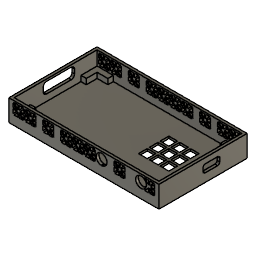
HomecurrentMoniter_BottomPlateHCM updated (Autodesk Fusion 360 design; units mm, degrees)
part number: 2026-06-16-14-03-26-042
Autodesk Fusion 360 part; units mm, degrees
note: some values were not read from the file. Set by a fixed rule: which sketch regions a step uses.
(part 1 of 2)
sketch "Sketch1" plane through (0, 0, 0) normal (0, 0, 1) x (1, 0, 0)
  line L0 (58.46, -118.98) -> (188.61, -118.98)
  line L1 (188.61, -118.98) -> (188.61, -46.12)
  line L2 (188.61, -46.12) -> (58.46, -46.12)
  line L3 (58.46, -46.12) -> (58.46, -118.98)
  line L4 (190.61, -121) -> (190.61, -44.12)
  line L5 (190.61, -44.12) -> (56.46, -44.12)
  line L6 (56.46, -44.12) -> (56.46, -120.98)
  line L7 (53.96, -123.48) -> (193.11, -123.48)
  line L8 (193.11, -123.48) -> (193.11, -41.62)
  line L9 (193.11, -41.62) -> (53.96, -41.62)
  line L10 (53.96, -41.62) -> (53.96, -123.48)
  line L11 (56.46, -44.12) -> (190.61, -44.12)
  line L12 (190.61, -44.12) -> (190.61, -121)
  line L13 (56.46, -120.98) -> (56.46, -44.12)
  line L14 (56.46, -44.12) -> (71.46, -44.12)
  line L15 (56.46, -59.12) -> (56.46, -44.12)
  line L16 (190.61, -44.12) -> (175.61, -44.12)
  line L17 (190.61, -59.12) -> (190.61, -44.12)
  line L18 (71.46, -120.98) -> (71.46, -115.98)
  line L19 (61.46, -105.98) -> (56.46, -105.98)
  line L20 (61.46, -115.98) -> (66.46, -115.98)
  line L21 (61.46, -110.98) -> (61.46, -115.98)
  line L22 (61.46, -110.98) -> (61.46, -105.98)
  line L23 (66.46, -115.98) -> (71.46, -115.98)
  line L24 (56.46, -120.98) -> (190.61, -120.98)
  line L25 (180.61, -115.98) -> (175.61, -115.98)
  line L26 (185.61, -115.98) -> (180.61, -115.98)
  line L27 (185.61, -105.98) -> (190.61, -105.98)
  line L28 (185.61, -110.98) -> (185.61, -115.98)
  line L29 (185.61, -110.98) -> (185.61, -105.98)
  line L30 (175.61, -120.98) -> (175.61, -115.98)
  line L31 (175.61, -44.12) -> (175.61, -49.12)
  line L32 (180.61, -49.12) -> (175.61, -49.12)
  line L33 (185.61, -49.12) -> (180.61, -49.12)
  line L34 (185.61, -54.12) -> (185.61, -49.12)
  line L35 (185.61, -54.12) -> (185.61, -59.12)
  line L36 (185.61, -59.12) -> (190.61, -59.12)
  line L37 (71.46, -44.12) -> (71.46, -49.12)
  line L38 (66.46, -49.12) -> (71.46, -49.12)
  line L39 (61.46, -49.12) -> (66.46, -49.12)
  line L40 (61.46, -54.12) -> (61.46, -49.12)
  line L41 (61.46, -54.12) -> (61.46, -59.12)
  line L42 (61.46, -59.12) -> (56.46, -59.12)
  point P0 (190.61, -120.98)
  point P1 (188.61, -118.98)
  point P2 (190.61, -120.98)
  dimension "d3" = 15
  dimension "d4" = 15
  dimension "d5" = 15
  dimension "d6" = 15
  dimension "d7" = 15
  dimension "d8" = 15
  constraint horizontal L11
  constraint vertical L12
  constraint vertical L13
  constraint horizontal L14
  constraint vertical L15
  constraint horizontal L16
  constraint vertical L17
  constraint vertical L18
  constraint horizontal L19
  constraint perpendicular L19 L22
  constraint perpendicular L18 L23
  constraint coincident L24 L30.start
  constraint perpendicular L24 L30
  constraint coincident L18.start L24
  constraint perpendicular L18 L24
  measures "d3" distance of L5.end L14.end
  measures "d4" distance of L5.end L15.start
  measures "d5" distance of L4.end L16.end
  measures "d6" distance of L4.end L17.start
  measures "d7" distance of L6.end L18.start
  measures "d8" distance of L6.end L19.end
extrude "Extrude1" add sketch "Sketch1" along normal blind 2 contours L0 L3 L18 L19 L20 L21 L22 L23 | L0 L3 L6 L13 L18 L19 L24 | L0 L1 L2 L3 L18 L19 L20 L21 L22 L23 L25 L26 L27 L28 L29 L30 L31 L32 L33 L34 L35 L36 L37 L38 L39 L40 L41 L42 | L0 L18 L24 L30 | L3 L6 L13 L19 L42 | L0 L1 L25 L26 L27 L28 L29 L30 | L0 L1 L4 L12 L24 L27 L30 | L2 L3 L5 L6 L11 L13 L14 L15 L37 L42 | L2 L3 L37 L38 L39 L40 L41 L42 | L1 L4 L12 L27 L36 | L2 L5 L11 L31 L37 | L1 L2 L31 L32 L33 L34 L35 L36 | L1 L2 L4 L5 L11 L12 L16 L17 L31 L36 | L7 L8 L9 L10
extrude "Extrude2" add sketch "Sketch1" along normal blind 30
extrude "Extrude3" add 1 faces at (145.8933, -42.4533, 30) along direction (0, 0, -1) blind 6
extrude "Extrude4" add sketch "Sketch1" along normal blind 7 contours L0 L3 L18 L19 L20 L21 L22 L23 | L0 L1 L25 L26 L27 L28 L29 L30 | L2 L3 L5 L6 L11 L13 L14 L15 L37 L42 | L2 L3 L37 L38 L39 L40 L41 L42 | L1 L2 L31 L32 L33 L34 L35 L36 | L1 L2 L4 L5 L11 L12 L16 L17 L31 L36
sketch "Sketch2" plane through (0, 0, 0) normal (0, 0, 1) x (1, 0, 0)
extrude "Extrude5" add sketch "Sketch1" along normal blind 7 contours L0 L3 L6 L13 L18 L19 L24
extrude "Extrude6" add sketch "Sketch1" along normal blind 7 contours L0 L1 L25 L26 L27 L28 L29 L30 | L0 L1 L4 L12 L24 L27 L30
sketch "Sketch3" plane through (193.11, 0, 0) normal (1, 0, 0) x (0, 1, 0)
  line L0 (-123.48, 0) -> (-41.62, 0)
  line L1 (-41.62, 0) -> (-41.62, 30)
  line L2 (-123.48, 30) -> (-123.48, 0)
  line L3 (-77.8135, 12.9716) -> (-71.4735, 12.9716)
  line L4 (-71.4735, 12.9716) -> (-77.8135, 12.9716)
  arc A0 (-77.8135, 12.9716) -> (-79.1135, 11.6716) centre (-77.8135, 11.6716) ccw
  arc A1 (-77.8135, 12.9716) -> (-79.1135, 11.6716) centre (-77.8135, 11.6716) ccw
  arc A2 (-70.1735, 11.6716) -> (-71.4735, 12.9716) centre (-71.4735, 11.6716) ccw
  arc A3 (-70.1735, 11.6716) -> (-71.4735, 12.9716) centre (-71.4735, 11.6716) ccw
  line L5 (-70.1735, 11.6716) -> (-70.1735, 11.1116)
  line L6 (-70.1735, 11.1116) -> (-70.1735, 11.1366)
  line L7 (-70.1735, 11.1366) -> (-70.1735, 11.1116)
  line L8 (-70.1735, 11.1116) -> (-70.1735, 11.1366)
  line L9 (-70.1735, 11.1366) -> (-70.1735, 11.3916)
  line L10 (-70.1735, 11.3916) -> (-70.1735, 11.6716)
  line L11 (-79.1135, 11.1116) -> (-79.1135, 11.6716)
  line L12 (-79.1135, 11.6716) -> (-79.1135, 11.3916)
  line L13 (-79.1135, 11.3916) -> (-79.1135, 11.1366)
  line L14 (-79.1135, 11.1366) -> (-79.1135, 11.1116)
  line L15 (-79.1135, 11.1116) -> (-79.1135, 11.1366)
  line L16 (-79.1135, 11.1366) -> (-79.1135, 11.1116)
  arc A4 (-79.1135, 11.1116) -> (-77.8135, 9.8116) centre (-77.8135, 11.1116) ccw
  arc A5 (-79.1135, 11.1116) -> (-77.8135, 9.8116) centre (-77.8135, 11.1116) ccw
  arc A6 (-71.4735, 9.8116) -> (-70.1735, 11.1116) centre (-71.4735, 11.1116) ccw
  arc A7 (-71.4735, 9.8116) -> (-70.1735, 11.1116) centre (-71.4735, 11.1116) ccw
  line L17 (-80.5, 15) -> (-68.9871, 15)
  line L18 (-66.9871, 13) -> (-66.9871, 9.8116)
  line L19 (-68.9871, 7.8116) -> (-80.5, 7.8116)
  line L20 (-82.5, 9.8116) -> (-82.5, 13)
  arc A8 (-66.9871, 13) -> (-68.9871, 15) centre (-68.9871, 13) ccw
  arc A9 (-68.9871, 7.8116) -> (-66.9871, 9.8116) centre (-68.9871, 9.8116) ccw
  arc A10 (-82.5, 9.8116) -> (-80.5, 7.8116) centre (-80.5, 9.8116) ccw
  arc A11 (-80.5, 15) -> (-82.5, 13) centre (-80.5, 13) ccw
  line L21 (-41.62, 30) -> (-123.48, 30)
  dimension "d24" = 2
  constraint horizontal L17
  constraint vertical L18
  constraint horizontal L19
  constraint vertical L20
  constraint tangent L17 A8
  constraint tangent L18 A8
  constraint tangent L18 A9
  constraint tangent L19 A9
  constraint equal A8 A9
  constraint tangent L19 A10
  constraint tangent L20 A10
  constraint equal A8 A10
  constraint tangent L17 A11
  constraint tangent L20 A11
  constraint equal A8 A11
  measures "d24" radius of A8
extrude "Extrude7" cut sketch "Sketch3" against normal up to surface (2.5 mm away) contours L17 L18 L19 L20 A8 A9 A10 A11
sketch "Sketch4" plane through (53.96, 0, 0) normal (-1, 0, 0) x (0, -1, 0)
  line L0 (41.62, 0) -> (123.48, 0)
  line L1 (123.48, 0) -> (123.48, 30)
  line L2 (41.62, 30) -> (41.62, 0)
  arc A0 (87.1797, 12.5216) -> (87.0797, 12.6216) centre (87.0797, 12.5216) ccw
  line L3 (87.1797, 10.4716) -> (87.1797, 12.5216)
  line L4 (87.3797, 10.4716) -> (87.1797, 10.4716)
  line L5 (87.3797, 10.4216) -> (87.3797, 10.4716)
  line L6 (88.3797, 10.4216) -> (87.3797, 10.4216)
  line L7 (88.3797, 10.3216) -> (88.3797, 10.4216)
  line L8 (88.3797, 9.5216) -> (88.3797, 10.3216)
  line L9 (85.3997, 9.5216) -> (88.3797, 9.5216)
  line L10 (85.3997, 9.5216) -> (85.3947, 9.5216)
  line L11 (85.3947, 9.5216) -> (85.2997, 9.5216)
  line L12 (84.7997, 9.5216) -> (85.2997, 9.5216)
  line L13 (84.7997, 9.5216) -> (84.7948, 9.5216)
  line L14 (84.7948, 9.5216) -> (84.6997, 9.5216)
  line L15 (84.1297, 9.5216) -> (84.6997, 9.5216)
  line L16 (84.1297, 9.5216) -> (84.1247, 9.5216)
  line L17 (84.1247, 9.5216) -> (84.0297, 9.5216)
  line L18 (83.5297, 9.5216) -> (84.0297, 9.5216)
  line L19 (83.5297, 9.5216) -> (83.5248, 9.5216)
  line L20 (83.5248, 9.5216) -> (83.4297, 9.5216)
  line L21 (82.8597, 9.5216) -> (83.4297, 9.5216)
  line L22 (82.8597, 9.5216) -> (82.8547, 9.5216)
  line L23 (82.8547, 9.5216) -> (82.7597, 9.5216)
  line L24 (82.2597, 9.5216) -> (82.7597, 9.5216)
  line L25 (82.2597, 9.5216) -> (82.2548, 9.5216)
  line L26 (82.2548, 9.5216) -> (82.1597, 9.5216)
  line L27 (81.5897, 9.5216) -> (82.1597, 9.5216)
  line L28 (81.5897, 9.5216) -> (81.5847, 9.5216)
  line L29 (81.5847, 9.5216) -> (81.4897, 9.5216)
  line L30 (80.9897, 9.5216) -> (81.4897, 9.5216)
  line L31 (80.9897, 9.5216) -> (80.9848, 9.5216)
  line L32 (80.9848, 9.5216) -> (80.8897, 9.5216)
  line L33 (80.3197, 9.5216) -> (80.8897, 9.5216)
  line L34 (80.3197, 9.5216) -> (80.3147, 9.5216)
  line L35 (80.3147, 9.5216) -> (80.2197, 9.5216)
  line L36 (79.7197, 9.5216) -> (80.2197, 9.5216)
  line L37 (79.7197, 9.5216) -> (79.7148, 9.5216)
  line L38 (79.7148, 9.5216) -> (79.6197, 9.5216)
  line L39 (79.0497, 9.5216) -> (79.6197, 9.5216)
  line L40 (79.0497, 9.5216) -> (79.0447, 9.5216)
  line L41 (79.0447, 9.5216) -> (78.9497, 9.5216)
  line L42 (78.4497, 9.5216) -> (78.9497, 9.5216)
  line L43 (78.4497, 9.5216) -> (78.4448, 9.5216)
  line L44 (78.4448, 9.5216) -> (78.3497, 9.5216)
  line L45 (77.7797, 9.5216) -> (78.3497, 9.5216)
  line L46 (77.7797, 9.5216) -> (77.7747, 9.5216)
  line L47 (77.7747, 9.5216) -> (77.6797, 9.5216)
  line L48 (77.1797, 9.5216) -> (77.6797, 9.5216)
  line L49 (77.1797, 9.5216) -> (77.1748, 9.5216)
  line L50 (77.1748, 9.5216) -> (77.0797, 9.5216)
  line L51 (76.5097, 9.5216) -> (77.0797, 9.5216)
  line L52 (76.5097, 9.5216) -> (76.5047, 9.5216)
  line L53 (76.5047, 9.5216) -> (76.4097, 9.5216)
  line L54 (75.9097, 9.5216) -> (76.4097, 9.5216)
  line L55 (75.9097, 9.5216) -> (75.9048, 9.5216)
  line L56 (75.9048, 9.5216) -> (75.8097, 9.5216)
  line L57 (75.2397, 9.5216) -> (75.8097, 9.5216)
  line L58 (75.2397, 9.5216) -> (75.2347, 9.5216)
  line L59 (75.2347, 9.5216) -> (75.1397, 9.5216)
  line L60 (74.6397, 9.5216) -> (75.1397, 9.5216)
  line L61 (74.6397, 9.5216) -> (74.6348, 9.5216)
  line L62 (74.6348, 9.5216) -> (74.5397, 9.5216)
  line L63 (73.9697, 9.5216) -> (74.5397, 9.5216)
  line L64 (73.9697, 9.5216) -> (73.9647, 9.5216)
  line L65 (73.9647, 9.5216) -> (73.8697, 9.5216)
  line L66 (73.3697, 9.5216) -> (73.8697, 9.5216)
  line L67 (73.3697, 9.5216) -> (73.3648, 9.5216)
  line L68 (73.3648, 9.5216) -> (73.2697, 9.5216)
  line L69 (70.3797, 9.5216) -> (73.2697, 9.5216)
  line L70 (70.3797, 9.5216) -> (70.3797, 10.3216)
  line L71 (70.3797, 10.3216) -> (70.3797, 10.4216)
  line L72 (70.3797, 10.4216) -> (71.3797, 10.4216)
  line L73 (71.3797, 10.3216) -> (71.3797, 10.4216)
  line L74 (71.3797, 10.3216) -> (71.4797, 10.3216)
  line L75 (71.4797, 10.3216) -> (71.4797, 10.4216)
  line L76 (71.5797, 10.4216) -> (71.4797, 10.4216)
  line L77 (71.5797, 10.4216) -> (71.5797, 12.5216)
  arc A1 (71.6797, 12.6216) -> (71.5797, 12.5216) centre (71.6797, 12.5216) ccw
  line L78 (87.0797, 12.6216) -> (71.6797, 12.6216)
  line L79 (68, 18.0438) -> (91, 18.0438)
  line L80 (94, 15.0438) -> (94, 11)
  line L81 (91, 8) -> (68, 8)
  line L82 (65, 11) -> (65, 15.0438)
  arc A2 (68, 18.0438) -> (65, 15.0438) centre (68, 15.0438) ccw
  arc A3 (94, 15.0438) -> (91, 18.0438) centre (91, 15.0438) ccw
  arc A4 (91, 8) -> (94, 11) centre (91, 11) ccw
  arc A5 (65, 11) -> (68, 8) centre (68, 11) ccw
  line L83 (123.48, 30) -> (41.62, 30)
  dimension "d31" = 3
  constraint horizontal L79
  constraint vertical L80
  constraint horizontal L81
  constraint vertical L82
  constraint tangent L79 A2
  constraint tangent L82 A2
  constraint tangent L79 A3
  constraint tangent L80 A3
  constraint equal A2 A3
  constraint tangent L81 A4
  constraint tangent L80 A4
  constraint equal A2 A4
  constraint tangent L81 A5
  constraint tangent L82 A5
  constraint equal A2 A5
  measures "d31" radius of A2
extrude "Extrude8" cut sketch "Sketch4" against normal up to surface (2.5 mm away) contours A0 L3 L4 L5 L6 L7 L8 L9 L10 L11 L12 L13 L14 L15 L16 L17 L18 L19 L20 L21 L22 L23 L24 L25 L26 L27 L28 L29 L30 L31 L32 L33 L34 L35 L36 L37 L38 L39 L40 L41 L42 L43 L44 L45 L46 L47 L48 L49 L50 L51 L52 L53 L54 L55 L56 L57 L58 L59 L60 L61 L62 L63 L64 L65 L66 L67 L68 L69 L70 L71 L72 L73 L74 L75 L76 L77 A1 L78 | L79 L80 L81 L82 A2 A3 A4 A5
extrude "Extrude9" cut 1 faces at (145.8933, -42.4533, 30) along direction (0, 0, -1) blind 8
extrude "Extrude10" cut 1 faces at (145.8933, -42.4533, 22) along direction (0, 0, -1) blind 2
sketch "Sketch6" plane through (0, -123.48, 0) normal (0, -1, 0) x (1, 0, 0)
  line L0 (193.11, 20) -> (53.96, 20)
  line L1 (53.96, 20) -> (53.96, 0)
  line L2 (53.96, 0) -> (193.11, 0)
  line L3 (193.11, 0) -> (193.11, 20)
  line L4 (56.46, 20) -> (190.61, 20)
  line L5 (190.61, 20) -> (190.61, 7)
  line L6 (190.61, 7) -> (175.61, 7)
  line L7 (175.61, 7) -> (175.61, 2)
  line L8 (175.61, 2) -> (71.46, 2)
  line L9 (71.46, 2) -> (71.46, 7)
  line L10 (71.46, 7) -> (56.46, 7)
  line L11 (56.46, 7) -> (56.46, 20)
  line L12 (174.61, 3) -> (72.46, 3)
  line L13 (72.46, 3) -> (72.46, 8)
  line L14 (72.46, 8) -> (57.46, 8)
  line L15 (57.46, 8) -> (57.46, 19)
  line L16 (57.46, 19) -> (189.61, 19)
  line L17 (189.61, 19) -> (189.61, 8)
  line L18 (189.61, 8) -> (174.61, 8)
  line L19 (174.61, 8) -> (174.61, 3)
  line L20 (57.46, 19) -> (62.96, 19)
  line L21 (62.96, 19) -> (62.96, 13.5)
  line L22 (62.96, 13.5) -> (57.46, 13.5)
  line L23 (57.46, 13.5) -> (57.46, 19)
  line L24 (57.46, 19) -> (62.96, 13.5)
  line L25 (62.46, 18.5) -> (62.46, 14.7071)
  line L26 (58.6671, 18.5) -> (62.46, 14.7071)
  line L27 (58.6671, 18.5) -> (62.46, 18.5)
  line L28 (61.7529, 14) -> (57.96, 14)
  line L29 (57.96, 14) -> (57.96, 17.7929)
  line L30 (57.96, 17.7929) -> (61.7529, 14)
  line L31 (57.96, 13) -> (57.96, 9.2071)
  line L32 (57.96, 9.2071) -> (61.7529, 13)
  line L33 (61.7529, 13) -> (57.96, 13)
  line L34 (58.6671, 8.5) -> (62.46, 12.2929)
  line L35 (62.46, 8.5) -> (62.46, 12.2929)
  line L36 (58.6671, 8.5) -> (62.46, 8.5)
  line L37 (62.96, 13.5) -> (57.46, 13.5)
  line L38 (62.96, 8) -> (62.96, 13.5)
  line L39 (67.2529, 18.5) -> (63.46, 14.7071)
  line L40 (63.46, 18.5) -> (63.46, 14.7071)
  line L41 (67.2529, 18.5) -> (63.46, 18.5)
  line L42 (67.96, 17.7929) -> (64.1671, 14)
  line L43 (67.96, 14) -> (67.96, 17.7929)
  line L44 (64.1671, 14) -> (67.96, 14)
  line L45 (64.1671, 13) -> (67.96, 13)
  line L46 (67.96, 13) -> (67.96, 9.2071)
  line L47 (67.96, 9.2071) -> (64.1671, 13)
  line L48 (67.2529, 8.5) -> (63.46, 12.2929)
  line L49 (63.46, 8.5) -> (63.46, 12.2929)
  line L50 (67.2529, 8.5) -> (63.46, 8.5)
  line L51 (68.46, 8) -> (68.46, 19)
  line L52 (78.2529, 18.5) -> (74.46, 18.5)
  line L53 (78.2529, 18.5) -> (74.46, 14.7071)
  line L54 (74.46, 18.5) -> (74.46, 14.7071)
  line L55 (78.96, 17.7929) -> (75.1671, 14)
  line L56 (78.96, 14) -> (78.96, 17.7929)
  line L57 (75.1671, 14) -> (78.96, 14)
  line L58 (75.1671, 13) -> (78.96, 13)
  line L59 (78.96, 13) -> (78.96, 9.2071)
  line L60 (78.96, 9.2071) -> (75.1671, 13)
  line L61 (74.46, 8.5) -> (74.46, 12.2929)
  line L62 (78.2529, 8.5) -> (74.46, 12.2929)
  line L63 (78.2529, 8.5) -> (74.46, 8.5)
  line L64 (68.96, 17.7929) -> (72.7529, 14)
  line L65 (69.6671, 18.5) -> (73.46, 18.5)
  line L66 (68.96, 9.2071) -> (72.7529, 13)
  line L67 (73.46, 18.5) -> (73.46, 14.7071)
  line L68 (68.96, 13) -> (68.96, 9.2071)
  line L69 (69.6671, 18.5) -> (73.46, 14.7071)
  line L70 (72.7529, 14) -> (68.96, 14)
  line L71 (68.96, 14) -> (68.96, 17.7929)
  line L72 (72.7529, 13) -> (68.96, 13)
  line L73 (73.46, 8.5) -> (73.46, 12.2929)
  line L74 (69.6671, 8.5) -> (73.46, 12.2929)
  line L75 (69.6671, 8.5) -> (73.46, 8.5)
  line L76 (123.535, 19) -> (123.535, 3)
  line L77 (123.535, 19) -> (57.46, 19)
  line L78 (119.2421, 13) -> (123.035, 13)
  line L79 (107.535, 18.5) -> (107.535, 14.7071)
  line L80 (111.3279, 8.5) -> (107.535, 12.2929)
  line L81 (117.535, 18.5) -> (117.535, 14.7071)
  line L82 (123.535, 19) -> (118.035, 13.5)
  line L83 (117.535, 8.5) -> (117.535, 12.2929)
  line L84 (123.035, 9.2071) -> (119.2421, 13)
  line L85 (118.035, 13.5) -> (123.535, 13.5)
  line L86 (123.535, 19) -> (118.035, 19)
  line L87 (122.3279, 8.5) -> (118.535, 8.5)
  line L88 (122.3279, 18.5) -> (118.535, 14.7071)
  line L89 (123.035, 17.7929) -> (119.2421, 14)
  line L90 (106.535, 8.5) -> (106.535, 12.2929)
  line L91 (111.3279, 18.5) -> (107.535, 14.7071)
  line L92 (118.035, 19) -> (118.035, 13.5)
  line L93 (118.535, 18.5) -> (118.535, 14.7071)
  line L94 (112.035, 14) -> (112.035, 17.7929)
  line L95 (123.535, 13.5) -> (123.535, 19)
  line L96 (112.035, 17.7929) -> (108.2421, 14)
  line L97 (112.035, 9.2071) -> (108.2421, 13)
  line L98 (108.2421, 13) -> (112.035, 13)
  line L99 (123.035, 13) -> (123.035, 9.2071)
  line L100 (111.3279, 8.5) -> (107.535, 8.5)
  line L101 (105.8279, 13) -> (102.035, 13)
  line L102 (102.7421, 8.5) -> (106.535, 8.5)
  line L103 (105.8279, 14) -> (102.035, 14)
  line L104 (102.7421, 8.5) -> (106.535, 12.2929)
  line L105 (102.7421, 18.5) -> (106.535, 18.5)
  line L106 (102.035, 9.2071) -> (105.8279, 13)
  line L107 (102.035, 13) -> (102.035, 9.2071)
  line L108 (102.035, 17.7929) -> (105.8279, 14)
  line L109 (102.7421, 18.5) -> (106.535, 14.7071)
  line L110 (118.535, 8.5) -> (118.535, 12.2929)
  line L111 (113.035, 14) -> (113.035, 17.7929)
  line L112 (122.3279, 8.5) -> (118.535, 12.2929)
  line L113 (111.3279, 18.5) -> (107.535, 18.5)
  line L114 (113.035, 17.7929) -> (116.8279, 14)
  line L115 (122.3279, 18.5) -> (118.535, 18.5)
  line L116 (119.2421, 14) -> (123.035, 14)
  line L117 (107.535, 8.5) -> (107.535, 12.2929)
  line L118 (113.035, 13) -> (113.035, 9.2071)
  line L119 (106.535, 18.5) -> (106.535, 14.7071)
  line L120 (123.035, 14) -> (123.035, 17.7929)
  line L121 (113.7421, 18.5) -> (117.535, 18.5)
  line L122 (118.035, 13.5) -> (123.535, 13.5)
  line L123 (108.2421, 14) -> (112.035, 14)
  line L124 (112.035, 13) -> (112.035, 9.2071)
  line L125 (113.7421, 18.5) -> (117.535, 14.7071)
  line L126 (116.8279, 13) -> (113.035, 13)
  line L127 (113.7421, 8.5) -> (117.535, 8.5)
  line L128 (116.8279, 14) -> (113.035, 14)
  line L129 (102.035, 14) -> (102.035, 17.7929)
  line L130 (113.035, 9.2071) -> (116.8279, 13)
  line L131 (113.7421, 8.5) -> (117.535, 12.2929)
  line L132 (90.4975, 19) -> (84.9975, 19)
  line L133 (84.9975, 19) -> (84.9975, 13.5)
  line L134 (84.9975, 13.5) -> (90.4975, 13.5)
  line L135 (90.4975, 13.5) -> (90.4975, 19)
  line L136 (84.9975, 19) -> (90.4975, 13.5)
  line L137 (84.9975, 19) -> (90.4975, 19)
  line L138 (89.9975, 14.7071) -> (89.9975, 18.5)
  line L139 (89.9975, 18.5) -> (86.2046, 18.5)
  line L140 (86.2046, 18.5) -> (89.9975, 14.7071)
  line L141 (85.4975, 14) -> (85.4975, 17.7929)
  line L142 (85.4975, 17.7929) -> (89.2904, 14)
  line L143 (89.2904, 14) -> (85.4975, 14)
  line L144 (86.2046, 8.5) -> (89.9975, 12.2929)
  line L145 (89.9975, 8.5) -> (86.2046, 8.5)
  line L146 (89.9975, 12.2929) -> (89.9975, 8.5)
  line L147 (85.4975, 9.2071) -> (89.2904, 13)
  line L148 (85.4975, 13) -> (85.4975, 9.2071)
  line L149 (89.2904, 13) -> (85.4975, 13)
  line L150 (95.4975, 17.7929) -> (91.7046, 14)
  line L151 (95.4975, 14) -> (95.4975, 17.7929)
  line L152 (94.7904, 18.5) -> (90.9975, 14.7071)
  line L153 (90.9975, 18.5) -> (94.7904, 18.5)
  line L154 (90.9975, 14.7071) -> (90.9975, 18.5)
  line L155 (95.4975, 9.2071) -> (91.7046, 13)
  line L156 (90.9975, 12.2929) -> (90.9975, 8.5)
  line L157 (94.7904, 8.5) -> (90.9975, 12.2929)
  line L158 (95.4975, 13) -> (95.4975, 9.2071)
  line L159 (90.9975, 8.5) -> (94.7904, 8.5)
  line L160 (91.7046, 13) -> (95.4975, 13)
  line L161 (91.7046, 14) -> (95.4975, 14)
  line L162 (79, 19) -> (84.9975, 19)
  line L163 (168.11, 17.7929) -> (171.9029, 14)
  line L164 (168.8171, 18.5) -> (172.61, 14.7071)
  line L165 (168.8171, 8.5) -> (172.61, 12.2929)
  line L166 (123.535, 19) -> (189.61, 19)
  line L167 (171.9029, 14) -> (168.11, 14)
  line L168 (168.8171, 8.5) -> (172.61, 8.5)
  line L169 (171.9029, 13) -> (168.11, 13)
  line L170 (168.8171, 18.5) -> (172.61, 18.5)
  line L171 (168.11, 9.2071) -> (171.9029, 13)
  line L172 (144.3279, 18.5) -> (140.535, 18.5)
  line L173 (178.11, 14) -> (178.11, 17.7929)
  line L174 (157.0725, 8.5) -> (160.8654, 8.5)
  line L175 (173.61, 8.5) -> (173.61, 12.2929)
  line L176 (184.61, 18.5) -> (184.61, 14.7071)
  line L177 (151.5725, 13) -> (151.5725, 9.2071)
  line L178 (145.035, 9.2071) -> (141.2421, 13)
  line L179 (189.61, 19) -> (184.11, 19)
  line L180 (145.035, 17.7929) -> (141.2421, 14)
  line L181 (189.61, 13.5) -> (189.61, 19)
  line L182 (151.5725, 17.7929) -> (155.3654, 14)
  line L183 (156.0725, 14.7071) -> (156.0725, 18.5)
  line L184 (145.035, 13) -> (145.035, 9.2071)
  line L185 (188.4029, 8.5) -> (184.61, 8.5)
  line L186 (189.11, 9.2071) -> (185.3171, 13)
  line L187 (188.4029, 8.5) -> (184.61, 12.2929)
  line L188 (124.7421, 8.5) -> (128.535, 12.2929)
  line L189 (124.035, 9.2071) -> (127.8279, 13)
  line L190 (129.035, 19) -> (129.035, 13.5)
  line L191 (135.7421, 18.5) -> (139.535, 14.7071)
  line L192 (156.5725, 19) -> (162.0725, 19)
  line L193 (135.035, 13) -> (135.035, 9.2071)
  line L194 (139.535, 18.5) -> (139.535, 14.7071)
  line L195 (130.2421, 13) -> (134.035, 13)
  line L196 (157.0725, 12.2929) -> (157.0725, 8.5)
  line L197 (140.535, 18.5) -> (140.535, 14.7071)
  line L198 (183.61, 18.5) -> (183.61, 14.7071)
  line L199 (134.035, 9.2071) -> (130.2421, 13)
  line L200 (134.035, 13) -> (134.035, 9.2071)
  line L201 (185.3171, 14) -> (189.11, 14)
  line L202 (129.535, 8.5) -> (129.535, 12.2929)
  line L203 (184.11, 8) -> (184.11, 13.5)
  line L204 (157.0725, 14.7071) -> (157.0725, 18.5)
  line L205 (184.61, 8.5) -> (184.61, 12.2929)
  line L206 (185.3171, 13) -> (189.11, 13)
  line L207 (135.035, 17.7929) -> (138.8279, 14)
  line L208 (188.4029, 18.5) -> (184.61, 14.7071)
  line L209 (183.61, 8.5) -> (183.61, 12.2929)
  line L210 (128.535, 8.5) -> (128.535, 12.2929)
  line L211 (189.11, 17.7929) -> (185.3171, 14)
  line L212 (179.8171, 8.5) -> (183.61, 12.2929)
  line L213 (144.3279, 8.5) -> (140.535, 8.5)
  line L214 (179.8171, 8.5) -> (183.61, 8.5)
  line L215 (182.9029, 14) -> (179.11, 14)
  line L216 (179.11, 9.2071) -> (182.9029, 13)
  line L217 (179.11, 17.7929) -> (182.9029, 14)
  line L218 (123.535, 19) -> (129.035, 19)
  line L219 (144.3279, 18.5) -> (140.535, 14.7071)
  line L220 (144.3279, 8.5) -> (140.535, 12.2929)
  line L221 (156.0725, 18.5) -> (152.2796, 18.5)
  line L222 (156.0725, 8.5) -> (152.2796, 8.5)
  line L223 (179.8171, 18.5) -> (183.61, 14.7071)
  line L224 (155.3654, 14) -> (151.5725, 14)
  line L225 (177.4029, 8.5) -> (173.61, 12.2929)
  line L226 (141.2421, 13) -> (145.035, 13)
  line L227 (156.0725, 12.2929) -> (156.0725, 8.5)
  line L228 (160.8654, 18.5) -> (157.0725, 14.7071)
  line L229 (123.535, 13.5) -> (123.535, 19)
  line L230 (129.035, 13.5) -> (123.535, 13.5)
  line L231 (162.0725, 19) -> (162.0725, 13.5)
  line L232 (172.61, 18.5) -> (172.61, 14.7071)
  line L233 (178.11, 9.2071) -> (174.3171, 13)
  line L234 (151.5725, 9.2071) -> (155.3654, 13)
  line L235 (129.035, 13.5) -> (123.535, 13.5)
  line L236 (177.4029, 18.5) -> (173.61, 18.5)
  line L237 (157.0725, 18.5) -> (160.8654, 18.5)
  line L238 (124.7421, 18.5) -> (128.535, 14.7071)
  line L239 (124.035, 14) -> (124.035, 17.7929)
  line L240 (130.2421, 14) -> (134.035, 14)
  line L241 (135.7421, 8.5) -> (139.535, 8.5)
  line L242 (129.535, 18.5) -> (129.535, 14.7071)
  line L243 (124.035, 17.7929) -> (127.8279, 14)
  line L244 (128.535, 18.5) -> (128.535, 14.7071)
  line L245 (135.035, 9.2071) -> (138.8279, 13)
  line L246 (135.7421, 8.5) -> (139.535, 12.2929)
  line L247 (127.8279, 14) -> (124.035, 14)
  line L248 (134.035, 14) -> (134.035, 17.7929)
  line L249 (135.035, 14) -> (135.035, 17.7929)
  line L250 (139.535, 8.5) -> (139.535, 12.2929)
  line L251 (138.8279, 14) -> (135.035, 14)
  line L252 (140.535, 8.5) -> (140.535, 12.2929)
  line L253 (133.3279, 18.5) -> (129.535, 18.5)
  line L254 (124.035, 13) -> (124.035, 9.2071)
  line L255 (152.2796, 8.5) -> (156.0725, 12.2929)
  line L256 (182.9029, 13) -> (179.11, 13)
  line L257 (155.3654, 13) -> (151.5725, 13)
  line L258 (123.535, 19) -> (129.035, 13.5)
  line L259 (157.7796, 14) -> (161.5725, 14)
  line L260 (145.035, 14) -> (145.035, 17.7929)
  line L261 (161.5725, 9.2071) -> (157.7796, 13)
  line L262 (179.8171, 18.5) -> (183.61, 18.5)
  line L263 (151.5725, 14) -> (151.5725, 17.7929)
  line L264 (141.2421, 14) -> (145.035, 14)
  line L265 (156.5725, 13.5) -> (156.5725, 19)
  line L266 (152.2796, 18.5) -> (156.0725, 14.7071)
  line L267 (157.7796, 13) -> (161.5725, 13)
  line L268 (133.3279, 8.5) -> (129.535, 12.2929)
  line L269 (173.61, 18.5) -> (173.61, 14.7071)
  line L270 (179.11, 13) -> (179.11, 9.2071)
  line L271 (161.5725, 14) -> (161.5725, 17.7929)
  line L272 (178.61, 8) -> (178.61, 19)
  line L273 (160.8654, 8.5) -> (157.0725, 12.2929)
  line L274 (161.5725, 17.7929) -> (157.7796, 14)
  line L275 (179.11, 14) -> (179.11, 17.7929)
  line L276 (177.4029, 8.5) -> (173.61, 8.5)
  line L277 (184.11, 13.5) -> (189.61, 13.5)
  line L278 (188.4029, 18.5) -> (184.61, 18.5)
  line L279 (133.3279, 8.5) -> (129.535, 8.5)
  line L280 (124.7421, 18.5) -> (128.535, 18.5)
  line L281 (127.8279, 13) -> (124.035, 13)
  line L282 (162.0725, 19) -> (156.5725, 13.5)
  line L283 (178.11, 13) -> (178.11, 9.2071)
  line L284 (189.61, 19) -> (184.11, 13.5)
  line L285 (138.8279, 13) -> (135.035, 13)
  line L286 (172.61, 8.5) -> (172.61, 12.2929)
  line L287 (162.0725, 13.5) -> (156.5725, 13.5)
  line L288 (174.3171, 14) -> (178.11, 14)
  line L289 (184.11, 13.5) -> (189.61, 13.5)
  line L290 (162.0725, 19) -> (156.5725, 19)
  line L291 (177.4029, 18.5) -> (173.61, 14.7071)
  line L292 (168.07, 19) -> (162.0725, 19)
  line L293 (168.11, 14) -> (168.11, 17.7929)
  line L294 (174.3171, 13) -> (178.11, 13)
  line L295 (189.11, 14) -> (189.11, 17.7929)
  line L296 (161.5725, 13) -> (161.5725, 9.2071)
  line L297 (133.3279, 18.5) -> (129.535, 14.7071)
  line L298 (134.035, 17.7929) -> (130.2421, 14)
  line L299 (178.11, 17.7929) -> (174.3171, 14)
  line L300 (189.11, 13) -> (189.11, 9.2071)
  line L301 (135.7421, 18.5) -> (139.535, 18.5)
  line L302 (184.11, 19) -> (184.11, 13.5)
  line L303 (124.7421, 8.5) -> (128.535, 8.5)
  line L304 (168.11, 13) -> (168.11, 9.2071)
  point P0 (112.535, 19)
  point P1 (134.535, 19)
  dimension "d58" = 1
  dimension "d59" = 5.5
  dimension "d60" = 5.5
  dimension "d61" = 0.5
  dimension "d62" = 0.5
  dimension "d63" = 5.5
  constraint horizontal L20
  constraint vertical L21
  constraint horizontal L22
  constraint vertical L23
  constraint symmetric L20.end L22 L38.start
  constraint symmetric L21.end L22 L24.end
  constraint symmetric L23.start L22 L37.end
  constraint symmetric L22 L25.start L35.start
  constraint symmetric L22 L25.end L34.end
  constraint symmetric L22 L26.start L34.start
  constraint symmetric L22 L28.start L32.end
  constraint symmetric L22 L28.end L31.start
  constraint symmetric L22 L29.end L31.end
  constraint symmetric L14.end L21 L51.start
  constraint symmetric L15.end L21 L51.end
  constraint symmetric L21 L25.start L40.start
  constraint symmetric L21 L25.end L39.end
  constraint symmetric L21 L26.start L39.start
  constraint symmetric L21 L28.start L42.end
  constraint symmetric L21 L28.end L43.start
  constraint symmetric L21 L29.end L42.start
  constraint symmetric L21 L31.start L45.end
  constraint symmetric L21 L31.end L46.end
  constraint symmetric L21 L32.end L45.start
  constraint symmetric L21 L34.start L48.start
  constraint symmetric L21 L34.end L48.end
  constraint symmetric L21 L35.start L49.start
  constraint symmetric L25.start L51 L52.end
  constraint symmetric L25.end L51 L53.end
  constraint symmetric L26.start L51 L52.start
  constraint symmetric L28.start L51 L55.end
  constraint symmetric L28.end L51 L56.start
  constraint symmetric L29.end L51 L55.start
  constraint symmetric L31.start L51 L58.end
  constraint symmetric L31.end L51 L59.end
  constraint symmetric L32.end L51 L58.start
  constraint symmetric L34.start L51 L62.start
  constraint symmetric L34.end L51 L61.end
  constraint symmetric L35.start L51 L61.start
  constraint symmetric L39.start L51 L65.start
  constraint symmetric L39.end L51 L67.end
  constraint symmetric L40.start L51 L65.end
  constraint symmetric L42.start L51 L64.start
  constraint symmetric L42.end L51 L64.end
  constraint symmetric L43.start L51 L70.end
  constraint symmetric L45.start L51 L66.end
  constraint symmetric L45.end L51 L68.start
  constraint symmetric L46.end L51 L66.start
  constraint symmetric L48.start L51 L74.start
  constraint symmetric L48.end L51 L73.end
  constraint symmetric L49.start L51 L73.start
  constraint midpoint L16 L76.start
  constraint midpoint L12 L76.end
  constraint midpoint L77 L132.start
  constraint horizontal L132
  constraint vertical L133
  constraint horizontal L134
  constraint vertical L135
  constraint perpendicular L138 L139
  constraint symmetric L136 L138.start L142.end
  constraint symmetric L136 L138.end L141.start
  constraint symmetric L136 L139.end L141.end
  constraint symmetric L134 L138.start L144.end
  constraint symmetric L134 L138.end L145.start
  constraint symmetric L134 L139.end L144.start
  constraint symmetric L134 L141.start L148.start
  constraint symmetric L134 L141.end L147.start
  constraint symmetric L134 L142.end L147.end
  constraint coincident L77 L162.start
  constraint symmetric L15.end L76 L16.end
  constraint symmetric L20.end L76 L179.end
  constraint symmetric L21.end L76 L203.end
  constraint symmetric L22.end L76 L181.start
  constraint symmetric L25.start L76 L176.start
  constraint symmetric L25.end L76 L176.end
  constraint symmetric L26.start L76 L208.start
  constraint symmetric L28.start L76 L201.start
  constraint symmetric L28.end L76 L201.end
  constraint symmetric L29.end L76 L211.start
  constraint symmetric L31.start L76 L206.end
  constraint symmetric L31.end L76 L186.start
  constraint symmetric L32.end L76 L186.end
  constraint symmetric L34.start L76 L185.start
  constraint symmetric L34.end L76 L187.end
  constraint symmetric L35.start L76 L185.end
  constraint symmetric L38.start L76 L203.start
  constraint symmetric L39.start L76 L223.start
  constraint symmetric L39.end L76 L198.end
  constraint symmetric L40.start L76 L198.start
  constraint symmetric L42.start L76 L217.start
  constraint symmetric L42.end L76 L215.start
  constraint symmetric L43.start L76 L215.end
  constraint symmetric L45.start L76 L216.end
  constraint symmetric L45.end L76 L256.end
  constraint symmetric L46.end L76 L216.start
  constraint symmetric L48.start L76 L212.start
  constraint symmetric L48.end L76 L209.end
  constraint symmetric L49.start L76 L209.start
  constraint symmetric L51.start L76 L272.start
  constraint symmetric L51.end L76 L272.end
  constraint symmetric L61.end L76 L165.end
  constraint symmetric L61.start L76 L168.end
  constraint symmetric L65.end L76 L236.end
  constraint symmetric L66.start L76 L233.start
  constraint symmetric L52.start L76 L164.start
  constraint symmetric L52.end L76 L170.end
  constraint symmetric L53.end L76 L164.end
  constraint symmetric L55.start L76 L163.start
  constraint symmetric L55.end L76 L163.end
  constraint symmetric L56.start L76 L167.end
  constraint symmetric L58.start L76 L169.start
  constraint symmetric L58.end L76 L169.end
  constraint symmetric L59.end L76 L171.start
  constraint symmetric L62.start L76 L165.start
  constraint symmetric L64.start L76 L173.end
  constraint symmetric L64.end L76 L288.start
  constraint symmetric L65.start L76 L236.start
  constraint symmetric L66.end L76 L233.end
  constraint symmetric L67.end L76 L269.end
  constraint symmetric L68.start L76 L283.start
  constraint symmetric L70.end L76 L173.start
  constraint symmetric L73.start L76 L175.start
  constraint symmetric L73.end L76 L175.end
  constraint symmetric L74.start L76 L225.start
  constraint symmetric L77.start L76 L82.start
  constraint symmetric L76 L132.start L192.start
  constraint symmetric L76 L80.start L241.start
  constraint symmetric L76 L100.end L241.end
  constraint symmetric L76 L85.end L95.start
  constraint symmetric L76 L83.start L202.start
  constraint symmetric L76 L83.end L202.end
  constraint symmetric L76 P0 P1
  constraint symmetric L76 L80.end L246.end
  constraint symmetric L76 L97.end L245.end
  constraint symmetric L76 L79.end L191.end
  constraint symmetric L76 L91.start L191.start
  constraint symmetric L76 L110.end L188.end
  constraint symmetric L76 L81.start L242.start
  constraint symmetric L76 L96.end L207.end
  constraint symmetric L76 L78.start L189.end
  constraint symmetric L76 L94.end L207.start
  constraint symmetric L76 L98.end L193.start
  constraint symmetric L76 L84.start L189.start
  constraint symmetric L76 L94.start L249.start
  constraint symmetric L76 L102.start L213.start
  constraint symmetric L76 L82.end L190.end
  constraint symmetric L76 L87.end L210.start
  constraint symmetric L76 L114.end L240.start
  constraint symmetric L76 L126.start L195.start
  constraint symmetric L76 L81.end L242.end
  constraint symmetric L76 L105.end L172.end
  constraint symmetric L76 L79.start L194.start
  constraint symmetric L76 L109.end L197.end
  constraint symmetric L76 L105.start L172.start
  constraint symmetric L76 L111.start L240.end
  constraint symmetric L76 L90.start L213.end
  constraint symmetric L76 L111.end L248.end
  constraint symmetric L76 L118.end L199.start
  constraint symmetric L76 L97.start L193.end
  constraint symmetric L76 L118.start L195.end
  constraint symmetric L76 L90.end L220.end
  constraint symmetric L76 L127.start L268.start
  constraint symmetric L76 L116.end L239.start
  constraint symmetric L76 L106.start L178.start
  constraint symmetric L76 L93.start L244.start
  constraint symmetric L76 L121.start L253.start
  constraint symmetric L76 L89.start L239.end
  constraint symmetric L76 L88.start L238.start
  constraint symmetric L76 L108.start L180.start
  constraint symmetric L76 L101.start L178.end
  constraint symmetric L76 L103.end L260.start
  constraint symmetric L76 L78.end L254.start
  constraint symmetric L76 L89.end L243.end
  constraint symmetric L76 L101.end L184.start
  constraint symmetric L76 L88.end L238.end
  constraint symmetric L76 L103.start L180.end
  constraint symmetric L76 L77.start L82.start
  constraint symmetric L76 L86.end L190.start
  constraint symmetric L76 L87.start L188.start
  constraint symmetric L76 L132.end L192.end
  constraint symmetric L76 L133.end L231.end
  constraint symmetric L76 L134.end L265.start
  constraint symmetric L76 L138.start L204.start
  constraint symmetric L76 L138.end L204.end
  constraint symmetric L76 L139.end L228.start
  constraint symmetric L76 L141.start L259.end
  constraint symmetric L76 L141.end L271.end
  constraint symmetric L76 L142.end L259.start
  constraint symmetric L76 L144.start L174.end
  constraint symmetric L76 L144.end L196.start
  constraint symmetric L76 L145.start L174.start
  constraint symmetric L76 L147.start L261.start
  constraint symmetric L76 L147.end L261.end
  constraint symmetric L76 L148.start L267.end
  constraint symmetric L76 L158.start L177.start
  constraint symmetric L76 L155.start L177.end
  constraint symmetric L76 L156.end L222.start
  constraint symmetric L76 L156.start L227.start
  constraint symmetric L76 L157.start L222.end
  constraint symmetric L76 L155.end L234.end
  constraint symmetric L76 L150.start L182.start
  constraint symmetric L76 L150.end L182.end
  constraint symmetric L76 L151.start L224.end
  constraint symmetric L76 L152.start L221.end
  constraint symmetric L76 L152.end L183.start
  constraint symmetric L76 L153.start L183.end
  constraint symmetric L76 L162.start L292.start
  measures "d59" distance of L15.end L20.end
  measures "d60" distance of L15.end L22.end
  measures "d63" distance of L132.start L132.end
sketch "Sketch7" plane through (0, -123.48, 0) normal (0, -1, 0) x (1, 0, 0)
  line L0 (138.9541, 9.4366) -> (140.6541, 9.4366)
  line L1 (175.8041, 9.4366) -> (177.5041, 9.4366)
  line L2 (135, 13.4903) -> (145, 13.4903)
  line L3 (145, 13.4903) -> (145, 8.5)
  line L4 (145, 8.5) -> (135, 8.5)
  line L5 (135, 8.5) -> (135, 13.4903)
  circle A0 centre (140, 13.4903) radius 5.0097
  circle A1 centre (176.5297, 13.4903) radius 5.0095
  dimension "d65" = 10.019
  constraint horizontal L2
  constraint vertical L3
  constraint horizontal L4
  constraint vertical L5
  constraint midpoint L2 A0.centre
  measures "d65" diameter of A1
extrude "Extrude11" cut sketch "Sketch7" against normal blind 4.5 contours L2 L3 L5 A0 | L2 L3 L4 L5 A0
extrude "Extrude12" cut sketch "Sketch7" against normal blind 4.5 contours A1
extrude "Extrude13" cut sketch "Sketch6" against normal blind 2.5 contours L25 L26 L27 | L28 L29 L30 | L31 L32 L33 | L34 L35 L36 | L39 L40 L41 | L42 L43 L44 | L45 L46 L47 | L48 L49 L50 | L52 L53 L54 | L55 L56 L57 | L58 L59 L60 | L61 L62 L63 | L64 L70 L71 | L65 L67 L69 | L66 L68 L72 | L73 L74 L75 | L78 L84 L99 | L79 L91 L113 | L80 L100 L117 | L81 L121 L125 | L83 L127 L131 | L87 L110 L112 | L88 L93 L115 | L89 L116 L120 | L90 L102 L104 | L94 L96 L123 | L97 L98 L124 | L101 L106 L107 | L103 L108 L129 | L105 L109 L119 | L111 L114 L128 | L118 L126 L130 | L138 L139 L140 | L141 L142 L143 | L144 L145 L146 | L147 L148 L149 | L150 L151 L161 | L152 L153 L154 | L155 L158 L160 | L156 L157 L159 | L174 L196 L273 | L176 L208 L278 | L177 L234 L257 | L182 L224 L263 | L183 L221 L266 | L185 L187 L205 | L186 L206 L300 | L188 L210 L303 | L189 L254 L281 | L195 L199 L200 | L198 L223 L262 | L201 L211 L295 | L202 L268 L279 | L204 L228 L237 | L209 L212 L214 | L222 L227 L255 | L238 L244 L280 | L239 L243 L247 | L240 L248 L298 | L242 L253 L297 | L259 L271 L274 | L261 L267 L296